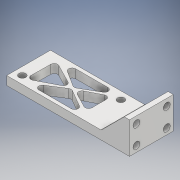
# Autodesk Inventor part: PingCover
Saved by Autodesk Inventor 2018.3 (Build 223284000, 284)
## iProperties
Created: 2018-08-21
Part Number: PingCover
Material: ABS プラスチック
Document SubType Name: Modeling
Designer: shun2
Density: 1.06 g/cm^3
Appearance: 滑らか - 白
Mass: 10.2262 g
Surface Area: 55.5665 cm^2
Volume: 9.6474 cm^3
Author: shun2
Autodesk Inventor part; units mm, degrees
ref_plane "YZ Plane" through (0, 0, 0) normal (1, 0, 0) x (0, 1, 0)
ref_plane "XZ Plane" through (0, 0, 0) normal (0, 1, 0) x (-1, 0, 0)
ref_plane "XY Plane" through (0, 0, 0) normal (0, 0, 1) x (1, 0, 0)
sketch "スケッチ2" plane through (0, 0, 0) normal (0, 0, 1) x (1, 0, 0)
  line L0 (22.85, 13.15) -> (-22.85, 13.15)
  line L1 (-22.85, 13.15) -> (-22.85, -8.15)
  line L2 (-22.85, -8.15) -> (22.85, -8.15)
  line L3 (22.85, -8.15) -> (22.85, 13.15)
  circle A0 centre (20.35, 10.65) radius 2
  circle A1 centre (-20.35, -5.65) radius 2
  circle A2 centre (12.2, 2.5) radius 8.15
  circle A3 centre (-12.2, 2.5) radius 8.15
  line L4 (-2.5, -13.15) -> (-2.5, -8.15)
  line L5 (0, -8.15) -> (0, -13.15)
  line L6 (2.5, -13.15) -> (2.5, -8.15)
  line L7 (-22.85, 15.15) -> (24.9059, 15.15)
  line L8 (-22.85, -10.15) -> (28.1108, -10.15)
  line L9 (-24.85, 8.1193) -> (-24.85, -10.15)
  line L10 (-24.85, 8.1193) -> (-24.85, 15.15)
  line L11 (-24.85, 15.15) -> (28.1108, 15.15)
  line L12 (28.1108, 15.15) -> (28.1108, -10.15)
  line L13 (28.1108, -10.15) -> (-24.85, -10.15)
  line L14 (-24.85, -10.15) -> (-24.85, 15.15)
  point P0 (0, 0)
  point P1 (0, 0)
  dimension "d24" = 25.3
  dimension "d55" = 4
  constraints: 30 end point, 6 perpendicular, 4 centre point, 3 horizontal, 3 parallel, 2 equal radius, 2 point on line, 1 midpoint, 1 vertical
  measures "d24" distance from line of L7.end L8
  measures "d55" diameter of A0
extrude "押し出し1" add sketch "スケッチ2" along normal blind 5 contours L3 L2 L1 L0 | L0 L1 L2 L4 L8 L13 L9 L10 L11 L7 L12 L6 L3 | L6 L8 L5 L2 | L2 L5 L8 L4 | A2 | A3
sketch "スケッチ7" plane through (0, 0, 0) normal (0, 0, -1) x (-1, 0, 0)
  line L0 (-28.1108, -10.15) -> (-28.1108, 15.15) projected
  line L1 (-28.1108, 15.15) -> (-43.1108, 15.15)
  line L2 (-43.1108, 15.15) -> (-43.1108, -10.15)
  line L3 (-43.1108, -10.15) -> (-28.1108, -10.15)
  line L4 (-28.1108, -10.15) -> (-28.1108, 15.15)
  point P0 (0, 0)
  dimension "d25" = 15
  constraints: 8 end point, 2 parallel, 1 horizontal, 1 perpendicular
  measures "d25" distance of L3.end L2.end
extrude "押し出し4" add sketch "スケッチ7" against normal blind 3.5
sketch "スケッチ8" plane through (0, 0, 0) normal (0, 0, -1) x (-1, 0, 0)
  line L0 (-43.1108, 15.15) -> (-43.1108, -10.15) projected
  line L1 (-43.1108, 15.15) -> (-46.1108, 15.15)
  line L2 (-46.1108, 15.15) -> (-46.1108, -10.15)
  line L3 (-46.1108, -10.15) -> (-43.1108, -10.15)
  line L4 (-43.1108, -10.15) -> (-43.1108, 15.15)
  point P0 (0, 0)
  dimension "d28" = 3
  constraints: 8 end point, 2 parallel, 1 horizontal, 1 perpendicular
  measures "d28" distance of L3.end L2.end
extrude "押し出し5" add sketch "スケッチ8" against normal blind 18.3
chamfer "面取り2" distance 14.8 angle 45 1 edges at (43.1108, 2.5, 3.5)
sketch "スケッチ9" plane through (46.1108, -10.15, 0) normal (1, 0, 0) x (0, 0, -1)
  line L0 (-18.3, 25.5) -> (-18.3, 0)
  line L1 (0, 0) -> (-18.3, 0)
  line L2 (0, 25.5) -> (0, 0)
  line L3 (-18.3, 25.5) -> (0, 25.5)
  line L4 (-18.3, 25.5) -> (-18.3, 0)
  line L5 (0, 0) -> (-18.3, 0)
  line L6 (0, 25.5) -> (0, 0)
  line L7 (-18.3, 25.5) -> (0, 25.5)
  line L8 (-18.3, 25.5) -> (-18.3, 0)
  line L9 (0, 0) -> (-18.3, 0)
  line L10 (0, 25.5) -> (0, 0)
  line L11 (-18.3, 25.5) -> (0, 25.5)
  line L12 (0, 25.3) -> (0, 0) projected
  line L13 (0, 25.3) -> (-18.3, 25.3) projected
  line L14 (-18.3, 0) -> (-18.3, 25.3) projected
  line L15 (0, 0) -> (-18.3, 0) projected
  circle A0 centre (-14.3, 4) radius 2
  circle A1 centre (-3.5, 4) radius 2
  circle A2 centre (-3.5, 21.5) radius 2
  circle A3 centre (-14.3, 21.5) radius 2
  point P0 (0, 10.15)
  dimension "d34" = 4
  dimension "d35" = 4
  dimension "d36" = 4
  dimension "d37" = 4
  constraints: 24 end point, 4 centre point
  measures "d34" diameter of A0
  measures "d35" diameter of A1
  measures "d36" diameter of A2
  measures "d37" diameter of A3
extrude "押し出し6" cut sketch "スケッチ9" against normal blind 12 contours A0 | A1 | A2 | A3
sketch "スケッチ10" plane through (0, 0, 5) normal (0, 0, 1) x (1, 0, 0)
  line L0 (28.1108, 15.15) -> (-24.85, 15.15) projected
  line L1 (-24.85, 15.15) -> (-24.85, -10.15) projected
  line L2 (-24.85, -10.15) -> (28.1108, -10.15) projected
  circle A0 centre (-20.35, -5.65) radius 2 projected
  circle A1 centre (20.35, 10.65) radius 2 projected
  line L3 (1.8215, 1.4851) -> (17.8805, 1.4851) construction
  line L4 (-0.4509, 3.7593) -> (-9.3797, 9.4181)
  line L5 (4.5361, 1.4851) -> (15.107, 1.4851) construction
  line L6 (-8.3091, 13.1074) -> (10.4211, 13.1074)
  line L7 (1.6197, 3.7165) -> (11.4211, 9.3754)
  line L8 (4.1627, 1.4851) -> (15.4804, 1.4851) construction
  arc A2 (11.4211, 9.3754) -> (10.4211, 13.1074) centre (10.4211, 11.1074) ccw
  arc A3 (-8.3091, 13.1074) -> (-9.3797, 9.4181) centre (-8.3091, 11.1074) ccw
  arc A4 (-0.4509, 3.7593) -> (1.6197, 3.7165) centre (0.6197, 5.4485) ccw
  line L9 (-0.4509, 1.2407) -> (-9.3797, -4.4181)
  line L10 (-8.3091, -8.1074) -> (10.4211, -8.1074)
  line L11 (1.6197, 1.2835) -> (11.4211, -4.3754)
  arc A5 (10.4211, -8.1074) -> (11.4211, -4.3754) centre (10.4211, -6.1074) ccw
  arc A6 (-9.3797, -4.4181) -> (-8.3091, -8.1074) centre (-8.3091, -6.1074) ccw
  arc A7 (1.6197, 1.2835) -> (-0.4509, 1.2407) centre (0.6197, -0.4485) ccw
  line L12 (-3.8471, 4.273) -> (-14.8005, 9.912)
  line L13 (-0.388, 2.4922) -> (11.9317, 2.4922) construction
  line L14 (-3.8493, 0.7155) -> (-14.9229, -4.9684)
  line L15 (-0.388, 2.4922) -> (12.0591, 2.4922) construction
  line L16 (-17.836, -3.1678) -> (-17.7158, 8.155)
  arc A8 (-3.8493, 0.7155) -> (-3.8471, 4.273) centre (-4.7626, 2.4948) ccw
  arc A9 (-14.8005, 9.912) -> (-17.7158, 8.155) centre (-15.7159, 8.1338) ccw
  arc A10 (-17.836, -3.1678) -> (-14.9229, -4.9684) centre (-15.8362, -3.1891) ccw
  line L17 (5.0865, 4.273) -> (13.0148, 8.3131)
  line L18 (5.0887, 0.7155) -> (13.0095, -3.3501)
  arc A11 (5.0865, 4.273) -> (5.0887, 0.7155) centre (6.002, 2.4948) ccw
  line L19 (15.9228, 6.5311) -> (15.9228, -1.5708)
  arc A12 (15.9228, 6.5311) -> (13.0148, 8.3131) centre (13.9228, 6.5311) ccw
  arc A13 (13.0095, -3.3501) -> (15.9228, -1.5708) centre (13.9228, -1.5708) ccw
  line L20 (28.1108, -10.15) -> (28.1108, 15.15) projected
  point P0 (0, 0)
  dimension "d49" = 2
  dimension "d54" = 2
  dimension "d57" = 2
  constraints: 34 end point, 24 point on circle, 16 tangent, 12 centre point, 6 horizontal, 5 equal radius, 4 equal length, 2 point on line, 1 vertical
  measures "d49" radius of A2
  measures "d54" radius of A8
  measures "d57" radius of A12
extrude "押し出し7" cut sketch "スケッチ10" against normal blind 12 contours L4 A3 L6 A2 L7 A4 | A7 L11 A5 L10 A6 L9 | A8 L14 A10 L16 A9 L12 | L17 A12 L19 A13 L18 A11
fillet "フィレット1" radius 2 3 edges at (28.1108, 2.5, 3.5) (28.1108, 2.5, 5) (28.3109, 2.5, 3.5)
sketch "スケッチ11" plane through (0, 0, 5) normal (0, 0, 1) x (1, 0, 0)
  line L0 (27.798, 15.15) -> (-24.85, 15.15) projected
  line L1 (-24.85, -10.15) -> (46.1108, -10.15) projected
  line L2 (27.798, 15.15) -> (30.798, 15.15)
  line L3 (30.798, 15.15) -> (30.798, -10.15)
  line L4 (30.798, -10.15) -> (27.798, -10.15)
  line L5 (27.798, -10.15) -> (27.798, 15.15)
  point P0 (0, 0)
  dimension "d61" = 3
  constraints: 8 end point, 2 parallel, 1 horizontal, 1 perpendicular, 1 point on line
  measures "d61" distance of L3.end L4.end
extrude "押し出し8" add sketch "スケッチ11" against normal blind 3
